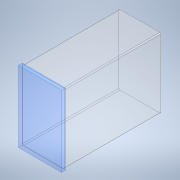
# Autodesk Inventor part: jar
Saved by Autodesk Inventor 2022 (Build 260153000, 153)
## iProperties
Created: 2022-08-22
Part Number: jar
Material: PMMA Plastic
Document SubType Name: Modeling
Designer: Sachin
Density: 1.188 g/cm^3
Appearance: Polycarbonate - Clear
Author: Sachin
Autodesk Inventor part; units mm, degrees
ref_plane "YZ Plane" through (0, 0, 0) normal (1, 0, 0) x (0, 1, 0)
ref_plane "XZ Plane" through (0, 0, 0) normal (0, 1, 0) x (-1, 0, 0)
ref_plane "XY Plane" through (0, 0, 0) normal (0, 0, 1) x (1, 0, 0)
sketch "Sketch1" plane through (0, 0, 0) normal (0, 0, 1) x (1, 0, 0)
  line L0 (0, -1.3086) -> (-76.2, -1.3086)
  line L1 (-76.2, -1.3086) -> (-76.2, 125.6914)
  line L2 (-76.2, 125.6914) -> (0, 125.6914)
  line L3 (0, 125.6914) -> (0, -1.3086)
  point P0 (0, 0)
  dimension "d0" = 76.2
  dimension "d1" = 127
  constraints: 8 end point, 2 parallel, 1 horizontal, 1 perpendicular
  measures "d0" distance of L0.start L0.end
  measures "d1" distance of L0.end L1.end
extrude "Extrusion1" add sketch "Sketch1" along normal blind 175
sketch "Sketch2" plane through (0, 0, 175) normal (0, 0, 1) x (1, 0, 0)
  line L0 (-77.1669, 127.1854) -> (1.3323, 127.1854)
  line L1 (1.3323, 127.1854) -> (1.3323, -2.5417)
  line L2 (1.3323, -2.5417) -> (-77.1669, -2.5417)
  line L3 (-77.1669, -2.5417) -> (-77.1669, 127.1854)
  point P0 (0, 0)
  constraints: 8 end point, 2 parallel, 1 horizontal, 1 perpendicular
extrude "Extrusion2" add sketch "Sketch2" along normal blind 7
fillet "Fillet1" radius 2 4 edges at (-76.2, -1.3086, 87.5) (0, -1.3086, 87.5) (-76.2, 125.6914, 87.5) (0, 125.6914, 87.5)
body "Solid1"
